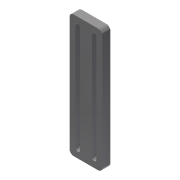
# Autodesk Inventor part: GARFO
Saved by Autodesk Inventor 2015 (Build 190159000, 159)
## iProperties
Created: 2016-08-09
Part Number: GARFO
Material: Aluminium AW-7020
Document SubType Name: Modeling
Designer: EriveltonDell
Density: 2.78 g/cm^3
Appearance: Stainless - Brushed
Mass: 1234.07 g
Surface Area: 731.335 cm^2
Volume: 443.911 cm^3
Author: EriveltonDell
Autodesk Inventor part; units mm, degrees
ref_plane "YZ Plane" through (0, 0, 0) normal (1, 0, 0) x (0, 1, 0)
ref_plane "XZ Plane" through (0, 0, 0) normal (0, 1, 0) x (-1, 0, 0)
ref_plane "XY Plane" through (0, 0, 0) normal (0, 0, 1) x (1, 0, 0)
sketch "Sketch5" plane through (0, 0, 0) normal (0, 1, 0) x (-1, 0, 0)
  line L0 (0, 0) -> (40, 0)
  line L1 (40, 0) -> (40, 150)
  line L2 (40, 150) -> (0, 150)
  line L3 (0, 150) -> (0, 0)
  line L4 (40, 150) -> (40, 140)
  line L5 (40, 140) -> (30, 140)
  circle A0 centre (30, 140) radius 2.75
  circle A1 centre (30, 10) radius 2.75
  circle A2 centre (10, 140) radius 2.75
  circle A3 centre (10, 10) radius 2.75
  line L6 (32.75, 140) -> (32.75, 10)
  line L7 (27.25, 10) -> (27.25, 140)
  line L8 (12.75, 140) -> (12.75, 10)
  line L9 (7.25, 10) -> (7.25, 140)
  dimension "d107" = 40
  dimension "d108" = 150
  dimension "d109" = 10
  dimension "d110" = 10
  dimension "d111" = 5.5
  dimension "d114" = 130
  dimension "d117" = 20
  constraints: 20 end point, 8 point on circle, 4 centre point, 4 tangent, 2 horizontal, 2 parallel, 2 perpendicular, 2 point on line, 1 coincident, 1 vertical, 6 other
  measures "d107" distance of L2.end L1.end
  measures "d108" distance of L1.end L0.end
  measures "d109" distance of L1.end L4.end
  measures "d110" distance of L4.end L5.end
  measures "d111" diameter of A0
  measures "d114" distance of A0.centre A1.centre
  measures "d117" distance of A0.centre A2.centre
extrude "Extrusion3" add sketch "Sketch5" along normal blind 10
sketch "Sketch6" plane through (0, 10, 0) normal (0, 1, 0) x (1, 0, 0)
  arc A0 (-32.75, -140) -> (-27.25, -140) centre (-30, -140) ccw projected
  circle A1 centre (-30, -140) radius 4.5
  arc A2 (-27.25, -10) -> (-32.75, -10) centre (-30, -10) ccw projected
  circle A3 centre (-30, -10) radius 4.5
  arc A4 (-7.25, -10) -> (-12.75, -10) centre (-10, -10) ccw projected
  circle A5 centre (-10, -10) radius 4.5
  circle A6 centre (-10, -140) radius 4.5
  line L0 (-34.5, -140) -> (-34.5, -10)
  line L1 (-25.5, -10) -> (-25.5, -140)
  line L2 (-14.5, -140) -> (-14.5, -10)
  line L3 (-5.5, -10) -> (-5.5, -140)
  point P0 (0, 0)
  dimension "d122" = 9
  dimension "d123" = 9
  dimension "d124" = 9
  dimension "d125" = 9
  constraints: 8 end point, 8 point on circle, 5 tangent, 4 centre point, 3 coincident
  measures "d122" diameter of A1
  measures "d123" diameter of A3
  measures "d124" diameter of A5
  measures "d125" diameter of A6
extrude "Extrusion4" cut sketch "Sketch6" against normal blind 6
fillet "Fillet2" radius 5 4 edges at (0, 5, 150) (-40, 5, 150) (0, 5, 0) (-40, 5, 0)
body "Solid3"
